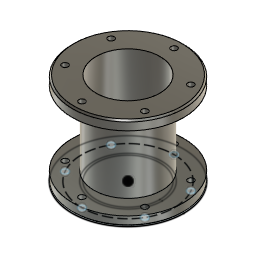
Component 4 (Autodesk Fusion 360 design; units mm, degrees)
Autodesk Fusion 360 part; units mm, degrees
sketch "Sketch1" plane through (0, 0, 0) normal (0, 0, 1) x (1, 0, 0)
  circle A0 centre (0, 0) radius 41.5
  circle A1 centre (0, 0) radius 72.5
  circle A2 centre (0, 0) radius 60 construction
  circle A3 centre (0, 0) radius 44.5
  circle A4 centre (0, 60) radius 4
  circle A5 centre (0, 0) radius 60 construction
  circle A6 centre (-51.9615, 30) radius 4
  circle A7 centre (0, 0) radius 60 construction
  circle A8 centre (-51.9615, -30) radius 4
  circle A9 centre (0, 0) radius 60 construction
  circle A10 centre (0, -60) radius 4
  circle A11 centre (0, 0) radius 60 construction
  circle A12 centre (51.9615, -30) radius 4
  circle A13 centre (0, 0) radius 60 construction
  circle A14 centre (51.9615, 30) radius 4
  dimension "d1" = 83
  dimension "d2" = 145
  dimension "d3" = 120
  dimension "d4" = 89
  dimension "d5" = 8
  dimension "d7" = 360
  constraint coincident A0.centre A1.centre
  constraint concentric A0 A1
  constraint concentric A1 A2
  constraint concentric A1 A3
  constraint coincident A2 A4.centre
  measures "d1" diameter of A0
  measures "d2" diameter of A1
  measures "d3" diameter of A2
  measures "d4" diameter of A3
  measures "d5" diameter of A4
extrude "Extrude1" add sketch "Sketch1" along normal blind 180 contours A0 makes body 1
extrude "Extrude2" add sketch "Sketch1" along normal blind 12 separate body contours A1 makes body 2
extrude "Extrude3" add sketch "Sketch1" along normal blind 12 separate body contours A3 makes body 3
extrude "Extrude4" cut sketch "Sketch1" along normal blind 385 contours A0 bodies 1
extrude "Extrude5" add sketch "Sketch1" along normal blind 120 contours A3 bodies 3 1 2
chamfer "Chamfer1" distance 2 angle 45 1 edges at (-67.5937, -26.2171, 0) on bodies 3
ref_plane "WorkPlane1" through (0, 0, 0) normal (0, -0.707107, 0.707107) x (1, 0, 0)
ref_plane "WorkPlane2" through (0, 0, 0) normal (-0.707107, 0, 0.707107) x (0.707107, 0, 0.707107)
ref_plane "WorkPlane3" through (0, 0, 0) normal (-0.707107, 0, 0.707107) x (0.707107, 0, 0.707107)
ref_plane "WorkPlane4" through (0, 0, 60) normal (0, 0, 1) x (1, 0, 0)
mirror "Mirror1" about plane through (0, 0, 60) normal (0, 0, 1) of bodies 3 merged
